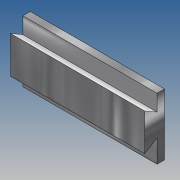
# Autodesk Inventor part: J008039
Saved by Autodesk Inventor 2018.3 (Build 223284000, 284)
## iProperties
Created: 2017-01-23
Material: ALUMINUM, 6061-T651
Vendor: HHMI: JRC - ID&F
Document SubType Name: Modeling
Designer: ARNOLDJ
Density: 2.7 g/cm^3
Appearance: Metal-AL-6061 (Machined)
Description: NEUROPIXELS GEN 2 DOVE TAIL MOUNT
Part Number: J008039
Project: COMMON
RuleStatus: InUse
AfterDocSave0: file://Part Number Cleaner
LAB/DEPT: APIG (SHARED RESOURCE)
REQUESTING SCIENTIST: HARRIS, TIM
SURFACE ROUGHNESS: 32 Ra
DESIGN DEPARTMENT: HHMI: JRC - ID&F
SPECIAL FINISH: NONE
ALTERED ITEM PART NUMBER: N/A
ALTERED ITEM VENDOR: N/A
ALTERED ITEM DESCRIPTION: N/A
Author: ARNOLDJ
Revision Number: 0
Autodesk Inventor part; units mm, degrees
ref_plane "YZ Plane" through (0, 0, 0) normal (1, 0, 0) x (0, 1, 0)
ref_plane "XZ Plane" through (0, 0, 0) normal (0, 1, 0) x (-1, 0, 0)
ref_plane "XY Plane" through (0, 0, 0) normal (0, 0, 1) x (1, 0, 0)
sketch "Sketch1" plane through (0, 0, 0) normal (0, 0, 1) x (1, 0, 0)
  line L0 (0, 2.3825) -> (0, -2.3825) projected
  line L1 (-5.7785, 0) -> (5.7785, 0) projected
  line L2 (4.1275, -1.7018) -> (-4.1275, -1.7018)
  line L3 (-4.1275, -1.7018) -> (-4.1275, 1.7018)
  line L4 (-4.1275, 1.7018) -> (4.1275, 1.7018)
  line L5 (4.1275, 1.7018) -> (4.1275, -1.7018)
  line L6 (4.1275, -1.7018) -> (-4.1275, 1.7018) construction
  line L7 (-4.1275, -1.7018) -> (4.1275, 1.7018) construction
  point P0 (0, 0)
  dimension "d0" = 8.255
  dimension "d1" = 3.4036
  constraints: 12 end point, 2 midpoint, 2 parallel, 1 horizontal, 1 perpendicular
  measures "d0" distance of L3.end L4.end
  measures "d1" distance of L2.end L3.end
extrude "Extrusion1" add sketch "Sketch1" along normal blind 1.2192
sketch "Sketch2" plane through (4.1275, -1.7018, 0) normal (1, 0, 0) x (0, 0, -1)
  line L0 (0, 0) -> (-1.2192, 0) projected
  line L1 (-1.2192, 0) -> (-1.2192, 3.4036) projected
  line L2 (0, 3.4036) -> (0, 0) projected
  line L3 (-0.4572, 0) -> (-0.4572, 1.0033)
  line L4 (-0.4572, 1.0033) -> (-1.2192, 0.5634)
  line L5 (-1.2192, 0.5634) -> (-1.2192, 0)
  line L6 (-1.2192, 0) -> (-0.4572, 0)
  line L7 (-1.463, 1.7018) -> (0.2438, 1.7018) projected
  point P0 (0, 1.7018)
  dimension "d6" = 60
  dimension "d15" = 0.5634
  dimension "d28" = 0.6985
  dimension "d32" = 1.1384
  dimension "d33" = 0.4572
  constraints: 8 end point, 2 perpendicular, 2 point on line, 1 collinear
  measures "d6" angle of L3 L4
  measures "d15" distance from line of L0 L4.end
  measures "d28" distance from line of L3.end L7
  measures "d32" distance from line of L7 L4.end
  measures "d33" distance between parallel lines of L3 L2
extrude "Extrusion2" cut sketch "Sketch2" against normal blind 8.255 contours L0 L1 L4 L3
mirror "Mirror1" about plane through (0, 0, 0) normal (0, 1, 0) of "Extrusion2"
sketch "Sketch5" plane through (-4.1275, 0, 0) normal (1, 0, 0) x (0, 1, 0)
  line L0 (1.7018, 0) -> (-1.7018, 0) projected
  line L1 (-1.7018, 0) -> (-1.7018, 0.4572) projected
  line L2 (1.7018, 0) -> (1.7018, 0.4572) projected
  line L3 (-1.7018, 0) -> (-2.0828, 0)
  line L4 (-2.0828, 0) -> (-2.0828, -0.3048)
  line L5 (-2.0828, -0.3048) -> (-1.7018, -0.3048)
  line L6 (-1.7018, -0.3048) -> (-1.7018, 0)
  line L7 (1.7018, 0) -> (2.0828, 0)
  line L8 (2.0828, 0) -> (2.0828, -0.3048)
  line L9 (2.0828, -0.3048) -> (1.7018, -0.3048)
  line L10 (1.7018, -0.3048) -> (1.7018, 0)
  line L11 (0, 1.524) -> (0, -0.6096) projected
  line L12 (-1.7018, 0.4572) -> (-2.0828, 0.4572)
  line L13 (-2.0828, 0.4572) -> (-2.0828, 0)
  point P0 (0, 0)
  dimension "d20" = 0.3048
  dimension "d29" = 0.381
  constraints: 20 end point, 4 parallel, 3 horizontal, 3 perpendicular, 1 collinear, 1 horizontal alignment, 1 point on line
  measures "d20" distance of L5.end L0.end
  measures "d29" distance of L4.end L5.end
extrude "Extrusion5" add sketch "Sketch5" along normal up to surface (8.255 mm away) contours L3 L13 L12 L1
extrude "Extrusion7" add sketch "Sketch5" along normal blind 4.826 contours L6 L5 L4 L3
body "Solid1"
